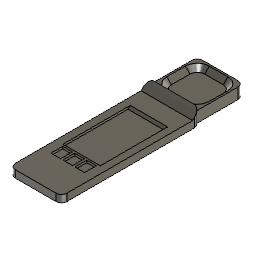
µPAD_tray (Autodesk Fusion 360 design; units mm, degrees)
part number: 2026-03-22-20-51-51-921
Autodesk Fusion 360 part; units mm, degrees
note: some values were not read from the file. Set by a fixed rule: which face or edge a step refers to.
sketch "Sketch1" plane through (0, 0, 0) normal (0, 0, 1) x (1, 0, 0)
  line L0 (-18.5263, 33.0877) -> (9.4737, 33.0877)
  line L1 (9.4737, 33.0877) -> (9.4737, -41.9123)
  line L2 (9.4737, -41.9123) -> (-18.5263, -41.9123)
  line L3 (-18.5263, -41.9123) -> (-18.5263, 33.0877)
  dimension "d1" = 28
  dimension "d2" = 75
  constraint horizontal L0
  constraint vertical L1
  constraint horizontal L2
  constraint vertical L3
  measures "d1" distance of L0.start L0.end
  measures "d2" distance of L0.start L2.end
extrude "Extrude1" add sketch "Sketch1" along normal blind 4
sketch "Sketch2" plane through (0, 0, 4) normal (0, 0, 1) x (-1, 0, 0)
  line L0 (18.5263, 41.9123) -> (-9.4737, 41.9123)
  line L1 (-9.4737, 41.9123) -> (-9.4737, -33.0877)
  line L2 (-9.4737, -33.0877) -> (18.5263, -33.0877)
  line L3 (18.5263, -33.0877) -> (18.5263, 41.9123)
  line L4 (14.5263, -18.0877) -> (-5.6737, -18.0877)
  line L5 (-5.6737, -18.0877) -> (-5.6737, 17.1123)
  line L6 (-5.6737, 17.1123) -> (14.5263, 17.1123)
  line L7 (14.5263, 17.1123) -> (14.5263, -18.0877)
  line L8 (10.8263, 18.1123) -> (7.6263, 18.1123)
  line L9 (7.6263, 18.1123) -> (7.6263, 21.3123)
  line L10 (7.6263, 21.3123) -> (10.8263, 21.3123)
  line L11 (10.8263, 21.3123) -> (10.8263, 18.1123)
  line L12 (6.1263, 18.1123) -> (2.9263, 18.1123)
  line L13 (2.9263, 18.1123) -> (2.9263, 21.3123)
  line L14 (2.9263, 21.3123) -> (6.1263, 21.3123)
  line L15 (6.1263, 21.3123) -> (6.1263, 18.1123)
  line L16 (1.4263, 18.1123) -> (-1.7737, 18.1123)
  line L17 (-1.7737, 18.1123) -> (-1.7737, 21.3123)
  line L18 (-1.7737, 21.3123) -> (1.4263, 21.3123)
  line L19 (1.4263, 21.3123) -> (1.4263, 18.1123)
  line L20 (18.5263, -33.0877) -> (-9.4737, -33.0877)
  line L21 (-9.4737, -33.0877) -> (-9.4737, -29.0877)
  line L22 (-9.4737, -29.0877) -> (18.5263, -29.0877)
  line L23 (18.5263, -29.0877) -> (18.5263, -33.0877)
  dimension "d5" = 20.2
  dimension "d6" = 35.2
  dimension "d7" = 15
  dimension "d8" = 4
  dimension "d9" = 3.2
  dimension "d10" = 3.2
  dimension "d11" = 1
  dimension "d12" = 3.2
  dimension "d13" = 3.2
  dimension "d14" = 3.2
  dimension "d15" = 3.2
  dimension "d16" = 1
  dimension "d17" = 1
  dimension "d18" = 12.4
  dimension "d19" = 1.5
  dimension "d20" = 1.5
  dimension "d23" = 28
  dimension "d24" = 4
  constraint horizontal L4
  constraint vertical L5
  constraint horizontal L6
  constraint vertical L7
  constraint horizontal L8
  constraint vertical L9
  constraint horizontal L10
  constraint vertical L11
  constraint horizontal L12
  constraint vertical L13
  constraint horizontal L14
  constraint vertical L15
  constraint horizontal L16
  constraint vertical L17
  constraint horizontal L18
  constraint vertical L19
  constraint horizontal L20
  constraint vertical L21
  constraint horizontal L22
  constraint vertical L23
  constraint coincident L2.end L3.start
  measures "d5" distance of L4.start L4.end
  measures "d6" distance of L4.start L6.end
  measures "d7" distance of L2 L4
  measures "d8" distance of L3 L7
  measures "d9" distance of L8.start L8.end
  measures "d10" distance of L8.start L10.end
  measures "d11" distance of L6 L8
  measures "d12" distance of L12.start L12.end
  measures "d13" distance of L12.start L14.end
  measures "d14" distance of L16.start L16.end
  measures "d15" distance of L16.start L18.end
  measures "d16" distance of L6 L12
  measures "d17" distance of L6 L16
  measures "d18" distance of L1 L13
  measures "d19" distance of L13 L19
  measures "d20" distance of L9 L15
  measures "d23" distance of L2.end L1.end
  measures "d24" distance of L2.end L22.end
extrude "Extrude2" cut sketch "Sketch2" against normal blind 1.2 contours L4 L5 L6 L7 | L8 L9 L10 L11 | L12 L13 L14 L15 | L16 L17 L18 L19
extrude "Extrude3" add sketch "Sketch2" along normal blind 4 contours L1 L2 L3 L20 L21 L22 L23
chamfer "Chamfer1" distance 4 angle 45 1 edges at (-4.5263, 29.0877, 8)
chamfer "Chamfer2" distance 1.2 angle 45 1 edges at (-4.4263, 18.0877, 4)
chamfer "Chamfer3" distance 1.2 angle 45 3 edges at (-9.2263, -21.3123, 4) (-4.5263, -21.3123, 4) (0.1737, -21.3123, 4)
sketch "Sketch3" plane through (0, 33.0877, 0) normal (0, 1, 0) x (-1, 0, 0)
  line L0 (-9.4737, 0) -> (18.5263, 0)
  line L1 (18.5263, 0) -> (18.5263, 8)
  line L2 (18.5263, 8) -> (-9.4737, 8)
  line L3 (-9.4737, 8) -> (-9.4737, 0)
  line L4 (-7.9737, 6) -> (17.0263, 6)
  line L5 (17.0263, 6) -> (17.0263, 0)
  line L6 (17.0263, 0) -> (-7.9737, 0)
  line L7 (-7.9737, 0) -> (-7.9737, 6)
  dimension "d30" = 25
  dimension "d31" = 6
  dimension "d32" = 2
  dimension "d33" = 1.5
  constraint horizontal L4
  constraint vertical L5
  constraint horizontal L6
  constraint vertical L7
  measures "d30" distance of L4.start L4.end
  measures "d31" distance of L4.start L6.end
  measures "d32" distance of L2 L4
  measures "d33" distance of L3 L7
extrude "Extrude4" add sketch "Sketch3" along normal blind 25 contours L0 L4 L5 L6 L7
sketch "Sketch4" plane through (0, 0, 6) normal (0, 0, 1) x (-1, 0, 0)
  line L0 (17.0263, -33.0877) -> (-7.9737, -33.0877)
  line L1 (-7.9737, -33.0877) -> (-7.9737, -58.0877)
  line L2 (-7.9737, -58.0877) -> (17.0263, -58.0877)
  line L3 (17.0263, -58.0877) -> (17.0263, -33.0877)
  line L4 (-0.4737, -36.5877) -> (9.5263, -36.5877)
  line L5 (13.5263, -40.5877) -> (13.5263, -50.5877)
  line L6 (9.5263, -54.5877) -> (-0.4737, -54.5877)
  line L7 (-4.4737, -50.5877) -> (-4.4737, -40.5877)
  arc A0 (-0.4737, -36.5877) -> (-4.4737, -40.5877) centre (-0.4737, -40.5877) ccw
  arc A1 (13.5263, -40.5877) -> (9.5263, -36.5877) centre (9.5263, -40.5877) ccw
  arc A2 (9.5263, -54.5877) -> (13.5263, -50.5877) centre (9.5263, -50.5877) ccw
  arc A3 (-4.4737, -50.5877) -> (-0.4737, -54.5877) centre (-0.4737, -50.5877) ccw
  point P0 (-4.4737, -36.5877)
  point P1 (13.5263, -36.5877)
  point P2 (-4.4737, -54.5877)
  dimension "d36" = 18
  dimension "d37" = 18
  dimension "d38" = 3.5
  dimension "d39" = 3.5
  dimension "d40" = 4
  constraint horizontal L4
  constraint vertical L5
  constraint horizontal L6
  constraint vertical L7
  constraint coincident P0 L4
  constraint coincident P0 L7
  constraint tangent L4 A0
  constraint tangent L7 A0
  constraint coincident P1 L4
  constraint coincident P1 L5
  constraint tangent L4 A1
  constraint tangent L5 A1
  constraint equal A0 A1
  constraint tangent L5 A2
  constraint tangent L6 A2
  constraint equal A0 A2
  constraint coincident P2 L6
  constraint coincident P2 L7
  constraint tangent L6 A3
  constraint tangent L7 A3
  constraint equal A0 A3
  measures "d36" distance of P0 P1
  measures "d37" distance of P0 P2
  measures "d38" distance of L1 L7
  measures "d39" distance of L2 L6
  measures "d40" radius of A0
extrude "Extrude5" cut sketch "Sketch4" against normal blind 2.5 contours L4 L5 L6 L7 A0 A1 A2 A3
chamfer "Chamfer4" distance 2.5 angle 45 8 edges at (4.4737, 45.5877, 6) (3.3021, 37.7593, 6) (-4.5263, 36.5877, 6) (-12.3548, 37.7593, 6) (-13.5263, 45.5877, 6) (-12.3548, 53.4161, 6) (-4.5263, 54.5877, 6) (3.3021, 53.4161, 6)
fillet "Fillet1" radius 3 2 edges at (-17.0263, 58.0877, 3) (7.9737, 58.0877, 3)
fillet "Fillet2" radius 3 2 edges at (-18.5263, 33.0877, 4) (9.4737, 33.0877, 4)
fillet "Fillet3" radius 3 2 edges at (-18.5263, -41.9123, 2) (9.4737, -41.9123, 2)
sketch "Sketch5" plane through (0, 33.0877, 0) normal (0, 1, 0) x (-1, 0, 0)
  line L0 (-6.4737, 8) -> (-6.4737, 6)
  line L1 (-6.4737, 6) -> (15.5263, 6)
  line L2 (15.5263, 6) -> (15.5263, 8)
  line L3 (15.5263, 8) -> (-6.4737, 8)
delete_face "DeleteFace1" 2 faces at (-8.693, -21.7122, 3.2002) (-8.693, -21.3123, 2.8002)
delete_face "DeleteFace2" 2 faces at (-3.993, -21.7122, 3.2002) (-3.993, -21.3123, 2.8002)
delete_face "DeleteFace3" 2 faces at (0.707, -21.7122, 3.2002) (0.707, -21.3123, 2.8002)
sketch "Sketch6" plane through (0, 0, 4) normal (0, 0, 1) x (-1, 0, 0)
  arc A0 (-6.4737, 41.9123) -> (-9.4737, 38.9123) centre (-6.4737, 38.9123) ccw
  line L0 (-9.4737, 38.9123) -> (-9.4737, -29.0877)
  line L1 (-9.4737, -29.0877) -> (18.5263, -29.0877)
  line L2 (18.5263, -29.0877) -> (18.5263, 38.9123)
  arc A1 (18.5263, 38.9123) -> (15.5263, 41.9123) centre (15.5263, 38.9123) ccw
  line L3 (15.5263, 41.9123) -> (-6.4737, 41.9123)
  line L4 (-5.6737, -19.2877) -> (-5.6737, 17.1123)
  line L5 (-5.6737, 17.1123) -> (14.5263, 17.1123)
  line L6 (14.5263, 17.1123) -> (14.5263, -19.2877)
  line L7 (14.5263, -19.2877) -> (-5.6737, -19.2877)
  line L8 (13.6263, 18.1123) -> (8.4263, 18.1123)
  line L9 (8.4263, 18.1123) -> (8.4263, 23.3123)
  line L10 (8.4263, 23.3123) -> (13.6263, 23.3123)
  line L11 (13.6263, 23.3123) -> (13.6263, 18.1123)
  line L12 (7.1263, 18.1123) -> (1.9263, 18.1123)
  line L13 (1.9263, 18.1123) -> (1.9263, 23.3123)
  line L14 (1.9263, 23.3123) -> (7.1263, 23.3123)
  line L15 (7.1263, 23.3123) -> (7.1263, 18.1123)
  line L16 (0.6263, 18.1123) -> (-4.5737, 18.1123)
  line L17 (-4.5737, 18.1123) -> (-4.5737, 23.3123)
  line L18 (-4.5737, 23.3123) -> (0.6263, 23.3123)
  line L19 (0.6263, 23.3123) -> (0.6263, 18.1123)
  dimension "d50" = 5.2
  dimension "d51" = 5.2
  dimension "d52" = 5.2
  dimension "d53" = 5.2
  dimension "d54" = 5.2
  dimension "d55" = 5.2
  dimension "d56" = 1
  dimension "d57" = 1
  dimension "d58" = 1
  dimension "d59" = 11.4
  dimension "d60" = 1.3
  dimension "d61" = 1.3
  constraint horizontal L8
  constraint vertical L9
  constraint horizontal L10
  constraint vertical L11
  constraint horizontal L12
  constraint vertical L13
  constraint horizontal L14
  constraint vertical L15
  constraint horizontal L16
  constraint vertical L17
  constraint horizontal L18
  constraint vertical L19
  measures "d50" distance of L8.start L8.end
  measures "d51" distance of L8.start L10.end
  measures "d52" distance of L12.start L12.end
  measures "d53" distance of L12.start L14.end
  measures "d54" distance of L16.start L16.end
  measures "d55" distance of L16.start L18.end
  measures "d56" distance of L5 L8
  measures "d57" distance of L5 L12
  measures "d58" distance of L5 L16
  measures "d59" distance of L0 L13
  measures "d60" distance of L9 L15
  measures "d61" distance of L13 L19
extrude "Extrude6" cut sketch "Sketch6" against normal blind 1.2 contours L8 L9 L10 L11 | L12 L13 L14 L15 | L16 L17 L18 L19
chamfer "Chamfer5" distance 1.2 angle 45 3 edges at (-4.5263, -23.3123, 4) (1.9737, -23.3123, 4) (-11.0263, -23.3123, 4)
equation "d59 = ( ( 28 - 5.2 ) / 2 ) * 1 mm"
